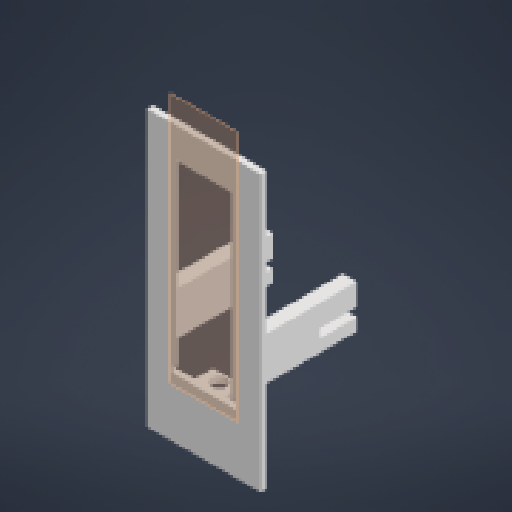
# Autodesk Inventor part: holderV2
Saved by Autodesk Inventor 2024.3 (Build 283343000, 343)
## iProperties
Created: 2025-08-18
Part Number: holderV2
Material: Generic
Document SubType Name: Modeling
Designer: giuseppe
Density: 1 g/cm^3
Appearance: Default
Author: giuseppe
## iProperties of the stored document holderV2_3DPrint.ipt
Created: 2025-08-20
Part Number: holderV2_3DPrint
Material: Generic
Document SubType Name: Modeling
Designer: giuseppe
Density: 1 g/cm^3
Appearance: Default
Author: giuseppe
Autodesk Inventor part; units mm, degrees
ref_plane "YZ Plane" through (0, 0, 0) normal (1, 0, 0) x (0, 1, 0)
ref_plane "XZ Plane" through (0, 0, 0) normal (0, 1, 0) x (-1, 0, 0)
ref_plane "XY Plane" through (0, 0, 0) normal (0, 0, 1) x (1, 0, 0)
ref_plane "Work Plane1" through (0, 0, 0) normal (0, 0, 1) x (1, 0, 0)
sketch "Sketch1" plane through (0, 0, 0) normal (0, 0, 1) x (1, 0, 0)
  line L0 (17.3205, 0) -> (17.3205, 45) projected
  line L1 (0, 0) -> (0, 45) projected
  line L2 (0, 0) -> (0, -13.8) projected
  line L3 (-1.3617, -13.8) -> (0, -13.8) projected
  line L4 (-1.3617, -15) -> (-1.3617, -13.8) projected
  line L5 (18.6822, -15) -> (-1.3617, -15) projected
  line L6 (18.6822, -13.8) -> (18.6822, -15) projected
  line L7 (17.3205, -13.8) -> (18.6822, -13.8) projected
  line L8 (17.3205, 0) -> (17.3205, -13.8) projected
  line L9 (27.3205, 55.5) -> (-10, 55.5)
  line L10 (-10, 55.5) -> (-10, -35)
  line L11 (-10, -35) -> (27.3205, -35)
  line L12 (27.3205, -35) -> (27.3205, 55.5)
  line L13 (-0.5, -13.3) -> (-0.5, 0)
  line L14 (-0.5, 0) -> (-0.5, 45.5)
  line L15 (-0.5, 45.5) -> (17.8205, 45.5)
  line L16 (17.8205, 45.5) -> (17.8205, 0)
  line L17 (17.8205, 0) -> (17.8205, -13.3)
  line L18 (17.8205, -13.3) -> (19.1822, -13.3)
  line L19 (19.1822, -13.3) -> (19.1822, -15.5)
  line L20 (19.1822, -15.5) -> (-1.8617, -15.5)
  line L21 (-1.8617, -15.5) -> (-1.8617, -13.3)
  line L22 (-1.8617, -13.3) -> (-0.5, -13.3)
  line L23 (17.3205, 45) -> (0, 45) projected
  dimension "d1" = 20
  dimension "d2" = 10
  dimension "d3" = 10
  dimension "d6" = 0.5
  dimension "d50" = 10
  dimension "d51" = 0.5
  dimension "d52" = 0.5
  constraints: 28 end point, 2 parallel, 1 horizontal, 1 perpendicular, 7 other
  measures "d1" distance between parallel lines of L11 L5
  measures "d2" distance between parallel lines of L10 L1
  measures "d3" distance between parallel lines of L0 L12
  measures "d6" distance between parallel lines of L2 L13
  measures "d50" distance between parallel lines of L9 L15
  measures "d51" distance between parallel lines of L1 L14
  measures "d52" distance between parallel lines of L15 L23
extrude "Extrusion1" add sketch "Sketch1" against normal blind 2 contours L12 L11 L10 L9
chamfer "Chamfer1" distance 1.36 angle 45 6 edges at (-0.5, -6.65, -2) (-0.5, 22.75, -2) (-1.8617, -14.4, -2) (17.8205, -6.65, -2) (17.8205, 22.75, -2) (19.1822, -14.4, -2)
sketch "Sketch2" plane through (-0.5, 45.5, 0) normal (0, -1, 0) x (1, 0, 0)
  circle A0 centre (9.1603, -5) radius 3.25 projected
  circle A1 centre (9.1603, -5) radius 3.05
  circle A2 centre (9.1603, -5) radius 4.25
  line L0 (27.8205, 0) -> (-9.5, 0) projected
  line L1 (27.8205, 0) -> (27.8205, -2) projected
  line L2 (-9.5, -2) -> (27.8205, -2) projected
  line L3 (-9.5, 0) -> (-9.5, -2) projected
  line L4 (13.0121, -6.7961) -> (15.2485, -2)
  line L5 (3.072, -2) -> (5.3084, -6.7961)
  line L6 (15.2485, -2) -> (3.072, -2)
  point P0 (0.5, 0)
  point P1 (9.7103, -2)
  point P2 (8.6103, -2)
  dimension "d10" = 0.2
  dimension "d11" = 1
  dimension "d12" = 65
  constraints: 6 end point, 2 centre point, 2 point on circle, 2 point on line, 2 tangent, 1 equal length, 1 parallel
  measures "d10" radial gap between concentric circles of A0 A1
  measures "d11" radial gap between concentric circles of A0 A2
  measures "d12" angle of L2 L4
extrude "Extrusion3" add sketch "Sketch2" along normal blind 2 contours A1 L2 picked at (10.1219, -5.0489)
sketch "Sketch3" plane through (-0.5, 45.5, 0) normal (0, 1, 0) x (1, 0, 0)
  circle A0 centre (9.1603, 5) radius 4.25 projected
  line L0 (3.072, 2) -> (5.3084, 6.7961) projected
  line L1 (-9.5, 2) -> (27.8205, 2) projected
  line L2 (13.0121, 6.7961) -> (15.2485, 2) projected
  point P0 (0.5, 0)
extrude "Extrusion4" add sketch "Sketch3" along normal blind 2 contours A0 L1 | A0 L2 L1 | A0 L1 L0 picked at (9.7449, 4.7598)
sketch "Sketch4" plane through (-1.8617, -15.5, 0) normal (0, 1, 0) x (1, 0, 0)
  circle A0 centre (10.522, 5) radius 2 projected
  line L0 (-8.1383, 2) -> (-1.36, 2) projected
  line L1 (-1.36, 2) -> (22.404, 2) projected
  line L2 (22.404, 2) -> (29.1822, 2) projected
  line L3 (29.1822, 2) -> (29.1822, 0) projected
  line L4 (29.1822, 0) -> (21.044, 0) projected
  line L5 (21.044, 0) -> (21.044, 0.64) projected
  line L6 (21.044, 0.64) -> (22.404, 2) projected
  line L7 (-8.1383, 0) -> (-8.1383, 2) projected
  line L8 (0, 0) -> (-8.1383, 0) projected
  line L9 (0, 0.64) -> (0, 0) projected
  line L10 (-1.36, 2) -> (0, 0.64) projected
  line L11 (21.044, 0) -> (0, 0) projected
  line L12 (5.522, 2) -> (5.522, 5)
  circle A1 centre (10.522, 5) radius 2.2
  line L13 (5.522, 5) -> (8.322, 5)
  line L14 (12.722, 5) -> (15.522, 5)
  line L15 (15.522, 5) -> (15.522, 2)
  point P0 (1.8617, 0)
  dimension "d19" = 0.2
  dimension "d20" = 10
  constraints: 8 end point, 4 horizontal alignment, 2 equal length, 2 point on circle, 2 point on line, 1 centre point, 1 perpendicular
  measures "d19" radial gap between concentric circles of A0 A1
  measures "d20" distance between parallel lines of L15 L12
extrude "Extrusion5" add sketch "Sketch4" against normal blind 2 contours L12 L13 A1 L14 L15 L1
ref_plane "Work Plane2" through (8.6603, -31, -5) normal (0, -1, 0) x (-1, 0, 0)
sketch "Sketch5" plane through (8.6603, -31, -5) normal (0, -1, 0) x (-1, 0, 0)
  circle A0 centre (0, 0) radius 3.5
  circle A1 centre (0, 0) radius 4.4
  point P0 (8.6603, -5)
  dimension "d23" = 0.9
  constraints: 2 centre point, 2 other
  measures "d23" radial gap between concentric circles of A0 A1
extrude "Extrusion6" cut sketch "Sketch5" along normal blind 0.75 and the other way blind 13.5 contours A0 | A1
sketch "Sketch8" plane through (-1.8617, -17.5, 0) normal (0, -1, 0) x (1, 0, 0)
  circle A0 centre (10.522, -5) radius 2.2
  arc A1 (12.722, -5) -> (8.322, -5) centre (10.522, -5) ccw projected
  line L0 (12.722, -5) -> (15.522, -5) projected
  line L1 (15.522, -5) -> (5.522, -5)
  line L2 (5.522, -5) -> (5.522, -8)
  line L3 (5.522, -8) -> (15.522, -8)
  line L4 (15.522, -8) -> (15.522, -5)
  line L5 (5.522, -2) -> (5.522, -5) projected
  point P0 (1.8617, 0)
  constraints: 8 end point, 2 collinear, 2 concentric, 2 parallel, 1 centre point, 1 horizontal, 1 perpendicular
extrude "Extrusion9" add sketch "Sketch8" against normal blind 2 contours L0 L4 L3 L2 L1 A0
sketch "Sketch9" plane through (0, 0, -2) normal (0, 0, -1) x (-1, 0, 0)
  line L0 (2.79, -0.65) -> (7.39, -0.65)
  line L1 (7.39, -0.65) -> (7.39, 6.55)
  line L2 (7.39, 6.55) -> (2.79, 6.55)
  line L3 (2.79, 6.55) -> (2.79, -0.65)
  line L4 (2.79, -3.55) -> (7.39, -3.55)
  line L5 (7.39, -3.55) -> (7.39, -7.65)
  line L6 (7.39, -7.65) -> (2.79, -7.65)
  line L7 (2.79, -7.65) -> (2.79, -3.55)
  line L8 (6.54, -3.35) -> (1.74, -3.35) construction
  line L9 (6.54, -0.85) -> (-23.86, -0.85) construction
  line L10 (2.59, -0.85) -> (2.59, 9.45) construction
  line L11 (2.59, -7.55) -> (2.59, -3.35) construction
  line L12 (-19.06, -3.35) -> (-23.86, -3.35) construction
  line L13 (6.54, -0.85) -> (-23.86, -0.85) construction
  line L14 (-19.91, -7.55) -> (-19.91, -3.35) construction
  line L15 (-19.91, -0.85) -> (-19.91, 9.45) construction
  line L16 (-24.71, -7.65) -> (-20.11, -7.65)
  line L17 (-20.11, -7.65) -> (-20.11, -3.55)
  line L18 (-20.11, -3.55) -> (-24.71, -3.55)
  line L19 (-24.71, -3.55) -> (-24.71, -7.65)
  line L20 (-24.71, -0.65) -> (-20.11, -0.65)
  line L21 (-20.11, -0.65) -> (-20.11, 6.55)
  line L22 (-20.11, 6.55) -> (-24.71, 6.55)
  line L23 (-24.71, 6.55) -> (-24.71, -0.65)
  line L24 (-19.81, -7.65) -> (-19.06, -7.65) projected
  line L25 (7.39, -3.35) -> (7.39, -0.85) projected
  line L26 (-24.71, -3.35) -> (-24.71, -0.85) projected
  point P0 (0, 0)
  dimension "d39" = 0.2
  dimension "d40" = 0.2
  dimension "d41" = 0.2
  dimension "d42" = 0.2
  dimension "d43" = 0.2
  dimension "d44" = 0.2
  dimension "d45" = 7.2
  constraints: 32 end point, 9 collinear, 8 parallel, 4 horizontal, 4 perpendicular
  measures "d39" distance between parallel lines of L11 L7
  measures "d40" distance between parallel lines of L8 L4
  measures "d41" distance between parallel lines of L9 L0
  measures "d42" distance between parallel lines of L14 L17
  measures "d43" distance between parallel lines of L12 L18
  measures "d44" distance between parallel lines of L9 L20
  measures "d45" distance of L22.end L20.start
ref_plane "Work Plane4" through (-6.54, -7.5503, -34.2) normal (0, 0, -1) x (0, 1, 0)
extrude "Extrusion10" add sketch "Sketch9" along normal up to surface (32.2 mm away)
sketch "Sketch10" plane through (0, 0, -2) normal (0, 0, -1) x (-1, 0, 0)
  line L0 (2.79, -7.65) -> (2.79, -3.55) projected
  line L1 (7.39, 6.55) -> (7.39, -0.65) projected
  line L2 (2.79, -3.55) -> (7.39, -3.55)
  line L3 (7.39, -3.55) -> (7.39, -0.65)
  line L4 (7.39, -0.65) -> (2.79, -0.65)
  line L5 (2.79, -0.65) -> (2.79, -3.55)
  line L6 (-20.11, -3.55) -> (-20.11, -7.65) projected
  line L7 (-20.11, -3.55) -> (-24.71, -3.55)
  line L8 (-24.71, -3.55) -> (-24.71, -0.65)
  line L9 (-24.71, -0.65) -> (-20.11, -0.65)
  line L10 (-20.11, -0.65) -> (-20.11, -3.55)
  line L11 (-24.71, -7.65) -> (-24.71, -3.55) projected
  point P0 (0, 0)
  constraints: 16 end point, 4 parallel, 2 horizontal, 2 perpendicular, 1 collinear, 1 point on line
extrude "Extrusion11" add sketch "Sketch10" along normal blind 19.8
sketch "Sketch12" plane through (-1.8617, -17.5, 0) normal (0, -1, 0) x (1, 0, 0)
  circle A0 centre (10.522, -5) radius 2.4
  circle A1 centre (10.522, -5) radius 2.2 projected
  point P0 (1.8617, 0)
  dimension "d53" = 0.2
  constraints: 1 centre point, 1 concentric
  measures "d53" radial gap between concentric circles of A0 A1
extrude "Extrusion12" cut sketch "Sketch12" against normal blind 19
body "Solid1"
